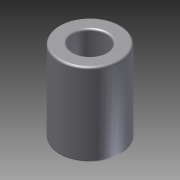
# Autodesk Inventor part: V5 Z Spacer
Saved by Autodesk Inventor 2012 (Build 160160000, 160)
## iProperties
Created: 2013-01-29
Part Number: V5 Z Spacer
Material: Default
Document SubType Name: Modeling
Designer: mce
Density: 1 g/cm^3
Mass: 2.70188 g
Surface Area: 16.4889 cm^2
Volume: 2.70188 cm^3
Author: mce
Autodesk Inventor part; units mm, degrees
ref_plane "YZ Plane" through (0, 0, 0) normal (1, 0, 0) x (0, 1, 0)
ref_plane "XZ Plane" through (0, 0, 0) normal (0, 1, 0) x (-1, 0, 0)
ref_plane "XY Plane" through (0, 0, 0) normal (0, 0, 1) x (1, 0, 0)
sketch "Sketch1" plane through (0, 0, 0) normal (0, 0, 1) x (1, 0, 0)
  circle A0 centre (0, 0) radius 7.45
  circle A1 centre (0, 0) radius 4
  dimension "d0" = 14.9
  dimension "d3" = 8
  constraints: 2 centre point, 2 coincident
  measures "d0" diameter of A0
  measures "d3" diameter of A1
extrude "Extrusion2" add sketch "Sketch1" along normal blind 20
fillet "Fillet1" radius 0.5 3 edges at (-7.45, 0, 0) (-7.45, 0, 20) (-4, 0, 20)
sketch "Sketch2" plane through (0, 0, 0) normal (0, 0, -1) x (-1, 0, 0)
  circle A0 centre (0, 0) radius 4 projected
  circle A1 centre (0, 0) radius 6.95 projected
  circle A2 centre (0, 0) radius 4
  constraints: 1 centre point, 1 coincident
extrude "Extrusion3" add sketch "Sketch2" against normal blind 4.5 contours A0
body "Solid2"
